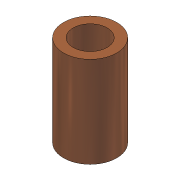
# Autodesk Inventor part: FOX-ME-117-03
Saved by Autodesk Inventor 2014 SP1 (Build 180222100, 222)
## iProperties
Created: 2011-03-09
Part Number: FOX-ME-117-03
Material: Copper 110H04
Document SubType Name: Modeling
Designer: Robert Davis
Mass: 0.76459 g
Surface Area: 2.21015 cm^2
Volume: 0.0857164 cm^3
Density: 8.92 g/cm^3
Description: CU SPACER FOR DELRIN
Appearance: Copper - Satin
Author: Robert Davis
Autodesk Inventor part; units mm, degrees
ref_plane "YZ Plane" through (0, 0, 0) normal (1, 0, 0) x (0, 1, 0)
ref_plane "XZ Plane" through (0, 0, 0) normal (0, 1, 0) x (-1, 0, 0)
ref_plane "XY Plane" through (0, 0, 0) normal (0, 0, 1) x (1, 0, 0)
sketch "Sketch1" plane through (0, 0, 0) normal (0, 0, 1) x (1, 0, 0)
  circle A0 centre (0, 0) radius 1.524
  circle A1 centre (0, 0) radius 2.3813
  dimension "d0" = 4.7625
  dimension "d1" = 3.048
  constraints: 2 centre point
  measures "d0" diameter of A1
  measures "d1" diameter of A0
extrude "Extrusion1" add sketch "Sketch1" along normal mid plane 8.15
body "Solid1"
